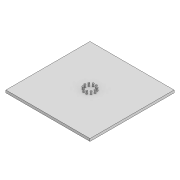
# Autodesk Inventor part: verify_geometry2
Saved by Autodesk Inventor 2021 (Build 250183000, 183)
## iProperties
Created: 2022-05-26
Part Number: verify_geometry2
Material: Generic
Document SubType Name: Modeling
Designer: Derm
Density: 1 g/cm^3
Appearance: Default
Author: Derm
Autodesk Inventor part; units mm, degrees
ref_plane "YZ Plane" through (0, 0, 0) normal (1, 0, 0) x (0, 1, 0)
ref_plane "XZ Plane" through (0, 0, 0) normal (0, 1, 0) x (-1, 0, 0)
ref_plane "XY Plane" through (0, 0, 0) normal (0, 0, 1) x (1, 0, 0)
sketch "Sketch1" plane through (0, 0, 0) normal (0, 1, 0) x (-1, 0, 0)
  line L0 (-50000, 50000) -> (50000, 50000)
  line L1 (50000, 50000) -> (50000, -50000)
  line L2 (50000, -50000) -> (-50000, -50000)
  line L3 (-50000, -50000) -> (-50000, 50000)
  line L4 (-50000, 50000) -> (50000, -50000) construction
  line L5 (50000, 50000) -> (-50000, -50000) construction
  point P0 (0, 0)
  dimension "d0" = 100000
  dimension "d1" = 100000
  constraints: 12 end point, 2 midpoint, 2 parallel, 1 horizontal, 1 perpendicular
  measures "d0" distance of L0.end L1.end
  measures "d1" distance of L1.end L2.end
extrude "Extrusion1" add sketch "Sketch1" against normal blind 3000
sketch "Sketch2" plane through (0, 0, 0) normal (0, 1, 0) x (1, 0, 0)
  circle A0 centre (0, 0) radius 6000 construction
  circle A1 centre (6000, -0.0911) radius 1000
  circle A2 centre (4854.1555, 3526.6379) radius 1000
  circle A3 centre (1854.1886, 5706.311) radius 1000
  circle A4 centre (-1854.0154, 5706.3672) radius 1000
  circle A5 centre (-4854.0484, 3526.7852) radius 1000
  circle A6 centre (-6000, 0.0911) radius 1000
  circle A7 centre (-4854.1555, -3526.6379) radius 1000
  circle A8 centre (-1854.1886, -5706.311) radius 1000
  circle A9 centre (1854.0154, -5706.3672) radius 1000
  circle A10 centre (4854.0484, -3526.7852) radius 1000
  dimension "d4" = 12000
  dimension "d5" = 2000
  dimension "d8" = 360
  constraints: 10 centre point, 1 coincident, 24 other
  measures "d5" diameter of A1
extrude "Extrusion2" add sketch "Sketch2" along normal blind 3000
body "Solid1"
